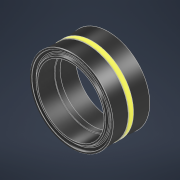
# Autodesk Inventor part: Uszczelka
Saved by Autodesk Inventor 2022 (Build 260153000, 153)
## iProperties
Created: 2023-04-12
Part Number: Uszczelka
Material: Ogólny
Document SubType Name: Modeling
Designer: jacek
Density: 1 g/cm^3
Appearance: Lśniąca — czarna
Author: jacek
Autodesk Inventor part; units mm, degrees
ref_plane "YZ Plane" through (0, 0, 0) normal (1, 0, 0) x (0, 1, 0)
ref_plane "XZ Plane" through (0, 0, 0) normal (0, 1, 0) x (-1, 0, 0)
ref_plane "XY Plane" through (0, 0, 0) normal (0, 0, 1) x (1, 0, 0)
sketch "Szkic1" plane through (0, 0, 0) normal (1, 0, 0) x (0, 1, 0)
  line L0 (0, 0) -> (0, -43.2297)
  line L1 (0, 0) -> (40, 0)
  line L2 (40, 0) -> (42, 0)
  line L3 (40, -46) -> (42, -46)
  line L4 (42, 0) -> (43, 0)
  line L5 (42, -46) -> (43, -46)
  line L6 (42, 0) -> (42.7721, -2.3162)
  line L7 (42, -46) -> (43, -43)
  line L8 (43.7208, -3) -> (45, -3)
  line L9 (43, -43) -> (45, -43)
  arc A0 (50, -1) -> (48.0279, -0.7656) centre (49, -1) ccw
  line L10 (49, 0) -> (42, 0)
  arc A1 (45, -3) -> (47.9102, -1.1114) centre (45, 0.1865) ccw
  arc A2 (47.9102, -1.1114) -> (48.0279, -0.7656) centre (46.0836, -0.2968) ccw
  line L11 (48.8421, -23) -> (49, -23)
  line L12 (50, -1) -> (49, -20)
  line L13 (49, -20) -> (39, -20)
  line L14 (39, -20) -> (39, -26)
  line L15 (39, -26) -> (49, -26)
  line L16 (40, 0) -> (40, -20)
  line L17 (40, -26) -> (40, -46)
  arc A3 (42.7721, -2.3162) -> (43.7208, -3) centre (43.7208, -2) ccw
  line L18 (42, -46) -> (43, -46)
  line L19 (42, -46) -> (42.7721, -43.6838)
  line L20 (43.7208, -43) -> (45, -43)
  arc A4 (48.0279, -45.2344) -> (50, -45) centre (49, -45) ccw
  line L21 (49, -46) -> (42, -46)
  arc A5 (47.9102, -44.8886) -> (45, -43) centre (45, -46.1865) ccw
  arc A6 (48.0279, -45.2344) -> (47.9102, -44.8886) centre (46.0836, -45.7032) ccw
  line L22 (50, -45) -> (49, -26)
  arc A7 (43.7208, -43) -> (42.7721, -43.6838) centre (43.7208, -44) ccw
  line L23 (49, -26) -> (49.5, -26)
  line L24 (49.5, -26) -> (49.5, -20)
  line L25 (49.5, -20) -> (49, -20)
  point P0 (43, -3)
  point P1 (42.386, -1.1581)
  point P2 (48.8441, -23)
  point P3 (42.386, -44.8419)
  dimension "d0" = 40
  dimension "d1" = 46
  dimension "d2" = 2
  dimension "d5" = 3
  dimension "d7" = 3
  dimension "d8" = 2
  dimension "d9" = 2
  dimension "d12" = 2
  dimension "d14" = 2
  dimension "d17" = 3
  dimension "d18" = 10
  dimension "d19" = 1
  constraints: 52 end point, 18 point on circle, 10 horizontal, 8 centre point, 8 point on line, 6 tangent, 4 perpendicular, 2 parallel, 1 collinear, 1 midpoint, 1 vertical
  measures "d0" distance of L0.start L1.end
  measures "d1" distance of L1.end L3.start
  measures "d2" distance of L1.end L2.end
  measures "d5" distance of L4.end point (43, -3)
  measures "d7" distance of L7.end L5.end
  measures "d8" distance of point (43, -3) L8.end
  measures "d9" distance of L7.end L9.end
  measures "d12" diameter of A0
  measures "d14" radius of A2
  measures "d17" distance of L11.end L12.end
  measures "d18" distance of L15.end L14.end
  measures "d19" radius of A3
revolve "Obrót1" add sketch "Szkic1" angle 360 about axis through (0, 0, 0) along (0, 0, -1) contours L2 L6 A3 L8 A1 A2 A0 L12 L13 L16 | L13 L25 L24 L23 L15 L14 | L15 L22 A4 A6 A5 L9 L7 L3 L17
